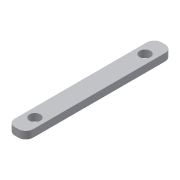
# Autodesk Inventor part: Halter_Verschraubung
Saved by Autodesk Inventor 2013 (Build 170138000, 138)
## iProperties
Created: 2013-07-02
Part Number: Halter_Verschraubung
Material: Allgemein
Document SubType Name: Modeling
Designer: Harald
Density: 1 g/cm^3
Author: Harald
Autodesk Inventor part; units mm, degrees
ref_plane "YZ Plane" through (0, 0, 0) normal (1, 0, 0) x (0, 1, 0)
ref_plane "XZ Plane" through (0, 0, 0) normal (0, 1, 0) x (-1, 0, 0)
ref_plane "XY Plane" through (0, 0, 0) normal (0, 0, 1) x (1, 0, 0)
sketch "Skizze1" plane through (0, 0, 0) normal (0, 0, 1) x (1, 0, 0)
  line L0 (2, 26) -> (3, 26)
  line L1 (5, 28) -> (5, 64)
  line L2 (3, 66) -> (2, 66)
  line L3 (0, 64) -> (0, 28)
  arc A0 (5, 64) -> (3, 66) centre (3, 64) ccw
  arc A1 (3, 26) -> (5, 28) centre (3, 28) ccw
  arc A2 (0, 28) -> (2, 26) centre (2, 28) ccw
  arc A3 (2, 66) -> (0, 64) centre (2, 64) ccw
  point P0 (0, 0)
  point P1 (0, 26)
  point P2 (5, 66)
  point P3 (5, 26)
  point P4 (0, 66)
  dimension "d0" = 5
  dimension "d1" = 40
  dimension "d2" = 2
  constraints: 8 end point, 8 point on circle, 8 point on line, 8 tangent, 4 centre point, 3 equal radius, 2 parallel, 1 horizontal, 1 perpendicular
  measures "d0" distance of point (0, 66) point (5, 66)
  measures "d1" distance of point (5, 66) point (5, 26)
  measures "d2" radius of A0
extrude "Extrusion1" add sketch "Skizze1" along normal blind 2
hole "Bohrung1" at (2.5, 61, 2) direction (0, 0, -1) diameter 3 end through all
hole "Bohrung2" at (2.5, 31, 2) direction (0, 0, -1) diameter 3 end through all
